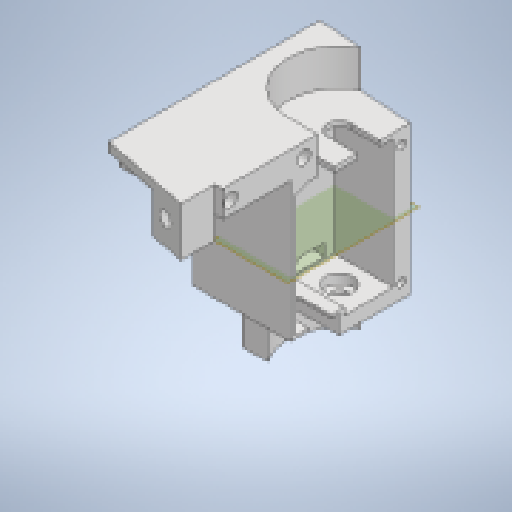
# Autodesk Inventor part: montaz_osi
Saved by Autodesk Inventor 2023.5 (Build 275446000, 446)
## iProperties
Created: 2025-03-26
Part Number: montaz_osi
Material: Ogólny
Document SubType Name: Modeling
Designer: kamil
Density: 1 g/cm^3
Appearance: Domyślna
Author: kamil
Autodesk Inventor part; units mm, degrees
ref_plane "YZ Plane" through (0, 0, 0) normal (1, 0, 0) x (0, 1, 0)
ref_plane "XZ Plane" through (0, 0, 0) normal (0, 1, 0) x (-1, 0, 0)
ref_plane "XY Plane" through (0, 0, 0) normal (0, 0, 1) x (1, 0, 0)
sketch "Szkic1" plane through (0, 0, 0) normal (0, 1, 0) x (-1, 0, 0)
  circle A0 centre (0, 0) radius 1.6
  line L0 (6, 6) -> (-6, 6)
  line L1 (-6, 6) -> (-6, -6)
  line L2 (-6, -6) -> (6, -6)
  line L3 (6, -6) -> (6, 6)
  line L4 (6, 6) -> (-6, -6) construction
  line L5 (-6, 6) -> (6, -6) construction
  dimension "d0" = 3.2
  dimension "d1" = 6
  dimension "d2" = 6
  constraints: 12 end point, 2 midpoint, 2 parallel, 1 centre point, 1 coincident, 1 horizontal, 1 perpendicular
  measures "d0" diameter of A0
  measures "d1" distance from line of L1 point (0, 0)
  measures "d2" distance from line of L2 point (0, 0)
extrude "Wyciągnięcie proste1" add sketch "Szkic1" along normal blind 1
sketch "Szkic2" plane through (0, 1, 0) normal (0, 1, 0) x (1, 0, 0)
  circle A0 centre (0, 0) radius 1.6 projected
  circle A1 centre (0, 0) radius 2.85
  line L0 (6, -6) -> (6, 6) projected
  line L1 (6, 6) -> (-6, 6) projected
  line L2 (-6, 6) -> (-6, -6) projected
  line L3 (-6, -6) -> (6, -6) projected
  circle A2 centre (0, 0) radius 1.6 projected
  dimension "d5" = 5.7
  constraints: 1 centre point, 1 coincident
  measures "d5" diameter of A1
extrude "Wyciągnięcie proste2" add sketch "Szkic2" along normal blind 2 contours L3 L2 L1 L0
sketch "Szkic3" plane through (-6, 0, 6) normal (0, 0, 1) x (1, 0, 0)
  line L0 (0, 0) -> (12, 0) projected
  line L1 (12, 0) -> (12, 3) projected
  line L2 (0, 3) -> (12, 3) projected
  line L3 (0, 0) -> (0, 3) projected
  point P0 (6, 0)
extrude "Wyciągnięcie proste3" cut sketch "Szkic3" against normal blind 1
sketch "Szkic4" plane through (-6, 0, -6) normal (-1, 0, 0) x (0, 0, 1)
  line L0 (21, 13.4099) -> (21, 27.4099) projected
  line L1 (1, 6.4099) -> (1, 20.4099) projected
  line L2 (11, 0) -> (11, 3) projected
  line L3 (0, 3) -> (11, 3) projected
  line L4 (0, 0) -> (0, 3) projected
  line L5 (0, 0) -> (11, 0) projected
  line L6 (20, 4.4099) -> (12, 4.4099) projected
  line L7 (2, 29.4099) -> (10, 29.4099) projected
  line L8 (1, 6.4099) -> (1, 3)
  line L9 (0, 3) -> (11, 3) projected
  line L10 (11, 3) -> (11, 4.4099)
  line L11 (11, 4.4099) -> (12, 4.4099)
  line L12 (1, 20.4099) -> (1, 29.4099)
  line L13 (1, 29.4099) -> (2, 29.4099)
  line L14 (1, 29.4099) -> (-2.5, 29.4099)
  line L15 (-2.5, 29.4099) -> (-2.5, 0)
  line L16 (11, 0) -> (0, 0) projected
  line L17 (-2.5, 0) -> (0, 0)
  line L18 (21, 13.4099) -> (21, 4.4099)
  line L19 (21, 4.4099) -> (20, 4.4099)
  line L20 (10, 29.4099) -> (11, 29.4099)
  line L21 (20.8, 28.4099) -> (11.2, 28.4099) projected
  line L22 (11, 29.4099) -> (11, 28.4099)
  line L23 (11, 28.4099) -> (11.2, 28.4099)
  line L24 (21, 27.4099) -> (21, 28.4099)
  line L25 (21, 28.4099) -> (20.8, 28.4099)
  point P0 (6, 0)
  dimension "d10" = 3.5
  constraints: 30 end point, 7 perpendicular, 4 point on line, 4 vertical, 1 collinear, 1 horizontal
  measures "d10" distance between parallel lines of L15 L1
extrude "Wyciągnięcie proste4" add sketch "Szkic4" along normal blind 2
sketch "Szkic5" plane through (-6, 0, -6) normal (1, 0, 0) x (0, 0, -1)
  line L0 (2.5, 29.4099) -> (2.5, 0) projected
  line L1 (-11, 29.4099) -> (2.5, 29.4099) projected
  line L2 (2.5, 0) -> (0, 0) projected
  line L3 (-11, 3) -> (0, 3) projected
  line L4 (-1, 21.4099) -> (-1, 20.4099) projected
  line L5 (-1, 28.4099) -> (-1, 29.4099) projected
  line L6 (-1, 21.4099) -> (-1, 28.4099)
  line L7 (-1, 20.4099) -> (-1, 0)
  line L8 (2.5, 0) -> (-11, 0) projected
  point P0 (-6, 0)
  constraints: 4 end point, 2 point on line, 1 vertical
extrude "Wyciągnięcie proste5" add sketch "Szkic5" along normal up to surface (12 mm away)
sketch "Szkic6" plane through (-8, 0, -6) normal (-1, 0, 0) x (0, 0, 1)
  line L0 (21, 4.4099) -> (21, 28.4099) projected
  line L1 (21, 4.4099) -> (22, 4.4099)
  line L2 (22, 4.4099) -> (22, 28.4099)
  line L3 (22, 28.4099) -> (21, 28.4099)
  line L4 (21, 28.4099) -> (21, 4.4099)
  line L5 (22, 31.9429) -> (22, -6.0571) projected
  point P0 (6, 0)
  dimension "d18" = 1
  constraints: 8 end point, 2 parallel, 1 horizontal, 1 perpendicular
  measures "d18" distance between parallel lines of L2 L0
extrude "Wyciągnięcie proste6" add sketch "Szkic6" against normal up to surface (14 mm away)
sketch "Szkic7" plane through (-8, 0, -6) normal (-1, 0, 0) x (0, 0, 1)
  line L0 (11, 0) -> (11, 4.4099) projected
  line L1 (11, 4.4099) -> (22, 4.4099) projected
  line L2 (22, 4.4099) -> (22, 28.4099) projected
  line L3 (22, 28.4099) -> (11, 28.4099) projected
  line L4 (11, 28.4099) -> (11, 29.4099) projected
  line L5 (11, 29.4099) -> (-2.5, 29.4099) projected
  line L6 (-2.5, 29.4099) -> (-2.5, 0) projected
  line L7 (-2.5, 0) -> (11, 0) projected
  line L8 (11, 28.4099) -> (22, 28.4099)
  line L9 (22, 28.4099) -> (22, 29.4099)
  line L10 (22, 29.4099) -> (11, 29.4099)
  line L11 (11, 29.4099) -> (11, 28.4099)
  line L12 (22, 4.4099) -> (22, 28.4099) projected
  point P0 (6, 0)
  constraints: 8 end point, 2 collinear, 2 parallel, 1 horizontal, 1 perpendicular
extrude "Wyciągnięcie proste7" add sketch "Szkic7" against normal up to surface (2 mm away) contours L3 L4 L10 L9
sketch "Szkic8" plane through (-6, 0, -6) normal (1, 0, 0) x (0, 0, -1)
  line L0 (-22, 28.4099) -> (-21, 28.4099) projected
  line L1 (-1, 29.4099) -> (-22, 29.4099) projected
  line L2 (-21, 4.4099) -> (-21, 28.4099) projected
  line L3 (-22, 29.4099) -> (-22, 28.4099) projected
  line L4 (-21, 28.4099) -> (-22, 28.4099)
  line L5 (-22, 28.4099) -> (-22, 29.4099)
  line L6 (-22, 29.4099) -> (-21, 29.4099)
  line L7 (-21, 29.4099) -> (-21, 28.4099)
  point P0 (-6, 0)
  constraints: 8 end point, 2 parallel, 1 horizontal, 1 perpendicular
extrude "Wyciągnięcie proste8" add sketch "Szkic8" along normal up to surface (12 mm away)
sketch "Szkic9" plane through (-8, 0, -6) normal (-1, 0, 0) x (0, 0, 1)
  line L0 (22, 29.4099) -> (-2.5, 29.4099) projected
  line L1 (22, 4.4099) -> (22, 29.4099) projected
  line L2 (16, 37.9429) -> (16, 29.9429) projected
  line L3 (16, 29.4099) -> (16, 29.9429)
  line L4 (22, 4.4099) -> (22, 29.4099) projected
  line L5 (22, 29.4099) -> (22, 37.9429)
  line L6 (22, 37.9429) -> (16, 37.9429)
  line L7 (16.5, 29.4099) -> (16.5, 29.9429)
  line L8 (16.5, 29.9429) -> (16.5, 37.4429)
  line L9 (16.5, 37.4429) -> (21.5, 37.4429)
  line L10 (21.5, 37.4429) -> (21.5, 29.4099)
  line L11 (21.5, 37.4429) -> (22, 37.4429)
  line L12 (16.5, 37.4429) -> (16.5, 37.9429)
  point P0 (6, 0)
  dimension "d23" = 0.5
  constraints: 18 end point, 4 perpendicular, 3 point on line, 2 vertical, 3 other
  measures "d23" distance between parallel lines of L6 L9
extrude "Wyciągnięcie proste9" add sketch "Szkic9" against normal up to surface (2 mm away) contours L0 L10 L11 L5 | L0 L7 L8 L9 L10 | L11 L9 L12 L6 L5
sketch "Szkic10" plane through (-6, 0, -6) normal (1, 0, 0) x (0, 0, -1)
  line L0 (-13.5, 29.9099) -> (-18.5, 29.9099) projected
  line L1 (-21, 4.4099) -> (-21, 29.4099) projected
  line L2 (-11, 4.4099) -> (-21, 4.4099) projected
  line L3 (-11, 3) -> (-11, 4.4099) projected
  line L4 (-1, 3) -> (-11, 3) projected
  line L5 (-1, 3) -> (-1, 29.4099) projected
  line L6 (-1, 29.4099) -> (-16.5, 29.4099) projected
  line L7 (-16.5, 29.4099) -> (-16.5, 37.9429) projected
  line L8 (-16.5, 37.9429) -> (-22, 37.9429) projected
  line L9 (-22, 37.9429) -> (-22, 29.4099) projected
  line L10 (-21, 29.4099) -> (-22, 29.4099) projected
  line L11 (-13.5, 30.4099) -> (-18.5, 30.4099)
  line L12 (-18.5, 30.4099) -> (-21, 29.4099)
  line L13 (-21, 29.4099) -> (-22, 29.4099) projected
  line L14 (-22, 29.4099) -> (-21, 29.4099)
  point P0 (-6, 0)
  point P1 (-16.5, 30.4099)
  dimension "d26" = 0.5
  constraints: 6 end point, 2 equal length, 1 vertical alignment
  measures "d26" distance between parallel lines of L0 L11
extrude "Wyciągnięcie proste10" add sketch "Szkic10" along normal up to surface (12 mm away) contours L10 L9 L8 L7 L11 L12
sketch "Szkic11" plane through (-8, 37.9429, 16) normal (0, 1, 0) x (1, 0, 0)
  circle A0 centre (8, 16) radius 10 projected
  circle A1 centre (8, 16) radius 10.5
  line L0 (0, 5.5) -> (14, 5.5) projected
  line L1 (0, 5.5) -> (2, 5.5) projected
  line L2 (2, 21) -> (2, 5.5) projected
  line L3 (2, 21) -> (14, 21) projected
  line L4 (14, 21) -> (14, 24.5) projected
  line L5 (14, 24.5) -> (0, 24.5) projected
  line L6 (0, 5.5) -> (0, 24.5) projected
  point P0 (8, 16)
  point P1 (8, 5.5)
  point P2 (0, 9.1993)
  constraints: 1 centre point, 1 tangent
extrude "Wyciągnięcie proste11" add sketch "Szkic11" against normal up to surface (7.533 mm away) contours L2 L0 L6 A1 | A1 L0 L2
sketch "Szkic12" plane through (-6, 30.4099, 10.5) normal (0, -1, 0) x (1, 0, 0)
  line L0 (0, -15.5) -> (0, 0) projected
  line L1 (-2, 0) -> (-2, -19) projected
  arc A0 (6, 0) -> (-2, -3.6993) centre (6, -10.5) ccw projected
  line L2 (-2, 0) -> (0, 0) projected
  point P0 (6, -10.5)
  point P1 (0, -1.8832)
extrude "Wyciągnięcie proste12" add sketch "Szkic12" along normal up to surface (1 mm away)
sketch "Szkic13" plane through (-6, 0, 5) normal (0, 0, 1) x (1, 0, 0)
  line L0 (12, 0) -> (-2, 0) projected
  line L1 (12, 3) -> (12, 0) projected
  line L2 (0, 3) -> (12, 3) projected
  line L3 (0, 3) -> (0, 4.4099) projected
  line L4 (0, 4.4099) -> (-2, 4.4099) projected
  line L5 (-2, 0) -> (-2, 4.4099) projected
  line L6 (12, 3) -> (12, 0) projected
  line L7 (-2, 0) -> (-2, 4.4099) projected
  line L8 (12, 0) -> (-2, 0)
  line L9 (-2, 0) -> (-2, 4.4099)
  line L10 (-2, 4.4099) -> (12, 4.4099)
  line L11 (12, 4.4099) -> (12, 0)
  point P0 (6, 0)
  constraints: 8 end point, 2 parallel, 1 horizontal, 1 perpendicular
extrude "Wyciągnięcie proste13" add sketch "Szkic13" along normal blind 1
sketch "Szkic14" plane through (-8, 4.4099, 16) normal (0, -1, 0) x (1, 0, 0)
  line L0 (0, -10) -> (0, 0) projected
  line L1 (0, 0) -> (14, 0) projected
  line L2 (14, -10) -> (2, -10) projected
  line L3 (0, -10) -> (2, -10) projected
  circle A0 centre (8, -6) radius 1.95 projected
  circle A1 centre (8, -6) radius 2.35
  line L4 (14, -10) -> (14, -2) projected
  line L5 (14, -1) -> (14, 0) projected
  line L6 (14, -2) -> (14, -1)
  line L7 (8, -8.35) -> (14, -8.35)
  line L8 (8, -3.65) -> (14, -3.65)
  line L9 (14, -5.5) -> (14, -3.5) projected
  point P0 (8, -16)
  point P1 (14, -3.65)
  dimension "d36" = 0.4
  constraints: 6 end point, 2 perpendicular, 2 point on circle, 2 point on line, 2 tangent, 1 centre point, 1 vertical
  measures "d36" radial gap between concentric circles of A0 A1
extrude "Wyciągnięcie proste14" add sketch "Szkic14" along normal blind 0.6 contours L0 L1 L5 L6 L4 L8 A1 L7 L2 L3
sketch "Szkic15" plane through (-8, 29.4099, -8.5) normal (0, 1, 0) x (1, 0, 0)
  circle A0 centre (8, -8.5) radius 1.95 projected
  circle A1 centre (8, -8.5) radius 2.35
  line L0 (0, -15.3007) -> (0, 0) projected
  line L1 (14, 0) -> (0, 0) projected
  line L2 (3, -13.5) -> (13, -13.5) projected
  line L3 (3, -15.5) -> (13, -15.5)
  line L4 (3, -15.5) -> (0, -15.5)
  line L5 (0, -15.5) -> (0, -15.3007)
  line L6 (14, -18.5) -> (14, 0) projected
  line L7 (13, -15.5) -> (14, -15.5)
  line L8 (13, -13.5) -> (14, -13.5)
  line L9 (8, -8.5) -> (8, -10.85)
  line L10 (8, -10.85) -> (14, -10.85)
  line L11 (8, -6.15) -> (14, -6.15)
  point P0 (8, -8.5)
  dimension "d39" = 0.4
  dimension "d40" = 2
  constraints: 16 end point, 5 perpendicular, 5 point on line, 2 point on circle, 1 centre point, 1 horizontal, 1 parallel, 1 tangent, 1 vertical
  measures "d39" radial gap between concentric circles of A0 A1
  measures "d40" distance between parallel lines of L2 L3
extrude "Wyciągnięcie proste15" add sketch "Szkic15" along normal blind 1 contours A1 L10 L6 L7 L3 L4 L5 L0 L1 L11
sketch "Szkic16" plane through (-7.8262, 29.4099, 7) normal (0, 1, 0) x (1, 0, 0)
  line L0 (1.8262, 0) -> (0, 0) projected
  arc A0 (0, 0) -> (1.8262, -1.6168) centre (7.8262, 7) ccw projected
  line L1 (1.8262, 0) -> (1.8262, -1.6168) projected
  point P0 (7.8262, 7)
extrude "Wyciągnięcie proste16" add sketch "Szkic16" along normal up to surface (1 mm away)
sketch "Szkic17" plane through (-8, 30.4099, -8.5) normal (0, 1, 0) x (1, 0, 0)
  circle A0 centre (8, -8.5) radius 10 projected
  circle A1 centre (8, -8.5) radius 10 projected
  circle A2 centre (8, -8.5) radius 9.5
  line L0 (14, -6.15) -> (14, 0) projected
  line L1 (14, 0) -> (0, 0) projected
  point P0 (8, -8.5)
  point P1 (12.2426, 0)
  point P2 (14, -1.1345)
  dimension "d45" = 0.5
  constraints: 1 centre point
  measures "d45" radial gap between concentric circles of A0 A2
sketch "Szkic18" plane through (6, 37.9429, 16) normal (1, 0, 0) x (0, 0, -1)
  line L0 (1, -8.533) -> (1, -33.533) projected
  line L1 (3.5, -7.533) -> (1, -8.533) projected
  line L2 (5.5, -7.533) -> (3.5, -7.533) projected
  line L3 (5.5, 0) -> (5.5, -7.533) projected
  line L4 (0, 0) -> (5.5, 0) projected
  line L5 (0, 0) -> (0, -34.133) projected
  line L6 (3.65, -34.133) -> (0, -34.133) projected
  line L7 (3.65, -33.533) -> (3.65, -34.133) projected
  line L8 (3.65, -33.533) -> (1, -33.533) projected
  point P0 (16, -37.9429)
  point P1 (2.75, -2.75)
  point P2 (2.75, 0)
  dimension "d48" = 2.75
  constraints: 1 midpoint, 1 vertical alignment
  measures "d48" distance from line of L4 point (2.75, -2.75)
hole "Otwór1" at (6, 35.1929, 13.25) direction (-1, 0, 0) diameter 2.8 end through all
ref_plane "Płaszczyzna konstrukcyjna1" through (0, 15.2049, 0) normal (0, -1, 0) x (1, 0, 0)
sketch "Szkic20" plane through (6, 3, 5) normal (1, 0, 0) x (0, 0, -1)
  line L0 (0, 0) -> (10, 0) projected
  line L1 (0, 0) -> (0, 1.4099) projected
  line L2 (0, 1.4099) -> (-2.65, 1.4099) projected
  line L3 (-2.65, 1.4099) -> (-2.65, 0.8099) projected
  line L4 (-1, 0.8099) -> (-2.65, 0.8099) projected
  line L5 (-1, -3) -> (-1, 0.8099) projected
  line L6 (-1, -3) -> (13.5, -3) projected
  line L7 (13.5, 27.4099) -> (13.5, -3) projected
  line L8 (7.35, 27.4099) -> (13.5, 27.4099) projected
  line L9 (7.35, 26.4099) -> (7.35, 27.4099) projected
  line L10 (7.35, 26.4099) -> (10, 26.4099) projected
  line L11 (10, 0) -> (10, 26.4099) projected
  line L12 (10, 26.4099) -> (13.5, 26.4099)
  line L13 (13.5, 27.4099) -> (13.5, -3) projected
  line L14 (0, 0) -> (10, 0) projected
  line L15 (10, 0) -> (10, -3)
  line L16 (-1, -3) -> (13.5, -3) projected
  line L17 (11.75, 26.4099) -> (11.75, -3)
  point P0 (5, -3)
  point P1 (11.75, 24.4099)
  point P2 (11.75, 0)
  dimension "d64" = 3
  dimension "d65" = 3
  constraints: 6 end point, 5 point on line, 3 perpendicular, 1 midpoint
  measures "d64" distance from line of point (11.75, 0) L6
  measures "d65" distance from line of L8 point (11.75, 24.41)
hole "Otwór3" at (6, 27.4099, -6.75) at (6, 3, -6.75) direction (-1, 0, 0) diameter 1.7 end through all
sketch "Szkic21" plane through (6, 37.9429, 16) normal (1, 0, 0) x (0, 0, -1)
  line L0 (-0.5, -5.5) -> (-13.5, -5.5) projected
  line L1 (-13.5, -44.5) -> (-0.5, -44.5) projected
  line L2 (-24, 0) -> (26, 0) projected
  line L3 (0, 0) -> (0, -34.133) projected
  line L4 (0, -5.5) -> (-14, -5.5)
  line L5 (-14, -5.5) -> (-14, 0)
  line L6 (-14, 0) -> (0, 0)
  line L7 (0, 0) -> (0, -5.5)
  line L8 (-14, -6) -> (-14, -44) projected
  point P0 (16, -37.9429)
  point P1 (-13.5, -5.5)
  constraints: 8 end point, 2 parallel, 2 point on line, 1 collinear, 1 horizontal, 1 perpendicular
extrude "Wyciągnięcie proste18" add sketch "Szkic21" against normal up to surface (14 mm away)
sketch "Szkic22" plane through (6, 30.4099, 10.5) normal (1, 0, 0) x (0, 0, -1)
  line L0 (-19.5, 1.533) -> (-19.5, -36.467) projected
  line L1 (-19.5, 2.033) -> (-5.5, 2.033) projected
  line L2 (-19.5, 7.533) -> (-19.5, 2.033) projected
  line L3 (-19.5, 1.533) -> (-19.5, 2.033)
  line L4 (-29.5, 7.533) -> (20.5, 7.533) projected
  line L5 (-29.5, -42.467) -> (-29.5, 7.533) projected
  line L6 (20.5, -42.467) -> (-29.5, -42.467) projected
  line L7 (20.5, 7.533) -> (20.5, -42.467) projected
  line L8 (-27.5, -40.467) -> (18.5, -40.467) projected
  line L9 (-27.5, 5.533) -> (-27.5, -40.467) projected
  line L10 (18.5, 5.533) -> (-27.5, 5.533) projected
  line L11 (18.5, -40.467) -> (18.5, 5.533) projected
  line L12 (-20.5, 7.533) -> (-20.5, -2.467)
  line L13 (-20.5, -2.467) -> (-19.5, -2.467)
  point P0 (10.5, -30.4099)
  point P1 (-20, -2.467)
  dimension "d75" = 1
  dimension "d76" = 10
  constraints: 6 end point, 2 point on line, 2 vertical, 1 midpoint, 1 perpendicular
  measures "d75" distance between parallel lines of L0 L12
  measures "d76" distance from line of L4 point (-20, -2.467)
extrude "Wyciągnięcie proste19" add sketch "Szkic22" against normal up to surface (14 mm away) contours L0 L13 L12 L10 L2 L3 | L10 L12 L4 L2
sketch "Szkic23" plane through (6, 30.4099, 10.5) normal (1, 0, 0) x (0, 0, -1)
  circle A0 centre (-2.75, 4.783) radius 1.4 projected
  line L0 (-4.5, -1) -> (-4.5, -26) projected
  line L1 (-2, 0) -> (-4.5, -1) projected
  line L2 (0, 0) -> (-2, 0) projected
  line L3 (0, 7.533) -> (0, 0) projected
  line L4 (0, 7.533) -> (-20.5, 7.533) projected
  line L5 (-20.5, 7.533) -> (-20.5, -2.467) projected
  line L6 (-20.5, -2.467) -> (-19.5, -2.467) projected
  line L7 (-19.5, -2.467) -> (-19.5, 2.033) projected
  line L8 (-19.5, 2.033) -> (-5.5, 2.033) projected
  line L9 (-5.5, 2.033) -> (-5.5, -26.6) projected
  line L10 (-1.85, -26.6) -> (-5.5, -26.6) projected
  line L11 (-1.85, -26) -> (-1.85, -26.6) projected
  line L12 (-1.85, -26) -> (-4.5, -26) projected
  point P0 (10.5, -30.4099)
  point P1 (-17.75, 4.783)
  dimension "d79" = 2.75
  dimension "d80" = 2.75
  constraints: 1 horizontal alignment
  measures "d79" distance from line of L4 point (-17.75, 4.783)
  measures "d80" distance from line of L5 point (-17.75, 4.783)
hole "Otwór4" at (6, 35.1929, 28.25) direction (-1, 0, 0) diameter 2.8 end through all
sketch "Szkic24" plane through (-8, 0, -6) normal (-1, 0, 0) x (0, 0, 1)
  circle A0 centre (17.5, 35.4429) radius 1.3 projected
  line L0 (37, 37.9429) -> (12.8007, 37.9429) projected
  line L1 (12.8007, 37.9429) -> (12.8007, 30.4099) projected
  line L2 (22.1993, 32.9429) -> (12.8007, 32.9429)
  line L3 (12.8007, 32.9429) -> (12.8007, 37.9429)
  line L4 (12.8007, 37.9429) -> (22.1993, 37.9429)
  line L5 (22.1993, 37.9429) -> (22.1993, 32.9429)
  line L6 (22.1993, 32.9429) -> (12.8007, 37.9429) construction
  line L7 (12.8007, 32.9429) -> (22.1993, 37.9429) construction
  line L8 (22, 32.4429) -> (22.1993, 32.9429)
  line L9 (36, 32.4429) -> (22, 32.4429) projected
  line L10 (22, 32.4429) -> (12.8007, 32.4429)
  point P0 (6, 0)
  constraints: 16 end point, 2 midpoint, 2 parallel, 2 perpendicular, 1 horizontal, 1 point on line
ref_plane "Płaszczyzna konstrukcyjna2" through (-15.1166, -12.0571, -10) normal (1, 0, 0) x (0, 1, 0)
ref_plane "Płaszczyzna konstrukcyjna3" through (-14, -12.0571, -10) normal (1, 0, 0) x (0, 1, 0)
extrude "Wyciągnięcie proste20" add sketch "Szkic24" along normal up to surface (6 mm away)
sketch "Szkic26" plane through (-8, 0, -6) normal (-1, 0, 0) x (0, 0, 1)
  line L0 (22, 32.4429) -> (12.8007, 32.4429) projected
  line L1 (12.8007, 32.4429) -> (12.8007, 30.4099) projected
  line L2 (-2.5, 30.4099) -> (12.8007, 30.4099) projected
  line L3 (-2.5, 0) -> (-2.5, 30.4099) projected
  line L4 (-2.5, 0) -> (12, 0) projected
  line L5 (12, 3.8099) -> (12, 0) projected
  line L6 (22, 3.8099) -> (12, 3.8099) projected
  line L7 (22, 3.8099) -> (22, 32.4429) projected
  circle A0 centre (-0.75, 27.4099) radius 0.85 projected
  circle A1 centre (-0.75, 3) radius 0.85 projected
  point P0 (6, 0)
extrude "Wyciągnięcie proste21" add sketch "Szkic26" along normal up to surface (6 mm away) contours L7 L6 L5 L4 L3 L2 L1 L0 | A0 | A1
sketch "Szkic27" plane through (-14, 0, -8.5) normal (-1, 0, 0) x (0, 0, 1)
  circle A0 centre (20, -9.5571) radius 1.3 projected
  line L0 (-1.5, -12.0571) -> (48.5, -12.0571) projected
  line L1 (24.5, 3.8099) -> (24.5, 32.4429) projected
  line L2 (0, 30.4099) -> (0, 0) projected
  line L3 (0, 0) -> (14.5, 0) projected
  line L4 (14.5, 0) -> (14.5, 3.8099) projected
  line L5 (14.5, 3.8099) -> (24.5, 3.8099) projected
  line L6 (15.3007, 37.9429) -> (15.3007, 30.4099) projected
  line L7 (15.3007, 0) -> (15.3007, -12.0571)
  line L8 (24.5, 32.4429) -> (24.5, 3.8099) projected
  line L9 (24.5, 3.8099) -> (24.5, -12.0571)
  line L10 (14.5, 0) -> (15.3007, 0)
  point P0 (8.5, 0)
  constraints: 6 end point, 2 collinear, 2 point on line, 1 horizontal, 1 perpendicular, 1 vertical
extrude "Wyciągnięcie proste22" add sketch "Szkic27" against normal blind 4
fillet "Zaokrąglenie1" radius 5 1 edges at (-10, 3.8099, 11)
sketch "Szkic28" plane through (0, 0, 0) normal (0, -1, 0) x (1, 0, 0)
  arc A0 (0, 10.5) -> (-8, 6.8007) centre (0, 0) ccw projected
  circle A1 centre (0, 0) radius 1.6 projected
  line L0 (6, 6) -> (6, -8.5) projected
  line L1 (6, 6) -> (-9.8563, 6) projected
  line L2 (-9.8563, 6.8007) -> (-9.8563, 6) projected
  line L3 (-14, 6.8007) -> (-9.8563, 6.8007) projected
  line L4 (-14, -8.5) -> (-14, 6.8007) projected
  line L5 (6, -8.5) -> (-14, -8.5) projected
  circle A2 centre (0, 0) radius 10.5
  point P0 (-6.1644, -8.5)
  point P1 (-8.6168, 6)
  constraints: 1 centre point, 1 coincident, 1 concentric
extrude "Wyciągnięcie proste23" add sketch "Szkic28" along normal up to surface (12.0571 mm away) contours A2 L5 L4 L3 L2 L1
sketch "Szkic29" plane through (-8, 30.4099, -8.5) normal (0, 1, 0) x (1, 0, 0)
  arc A0 (0, -15.3007) -> (2, -17.1168) centre (8, -8.5) ccw projected
  line L0 (2, -15.5) -> (2, -17.1168) projected
  line L1 (2, -15.5) -> (14, -15.5) projected
  line L2 (14, -15.5) -> (14, -10.85) projected
  line L3 (14, -10.85) -> (8, -10.85) projected
  arc A1 (8, -6.15) -> (8, -10.85) centre (8, -8.5) ccw projected
  line L4 (8, -6.15) -> (14, -6.15) projected
  line L5 (14, -6.15) -> (14, 0) projected
  line L6 (14, 0) -> (-6, 0) projected
  line L7 (-6, -15.3007) -> (-6, 0) projected
  line L8 (0, -15.3007) -> (-6, -15.3007) projected
  arc A2 (0, -15.3007) -> (8, -19) centre (8, -8.5) ccw projected
  circle A3 centre (8, -8.5) radius 10.5
  point P0 (8, -8.5)
  point P1 (1.8356, 0)
  constraints: 1 coincident, 3 other
extrude "Wyciągnięcie proste24" add sketch "Szkic29" along normal up to surface (7.533 mm away) contours L8 L7 L6 A3
sketch "Szkic30" plane through (6, 3, 5) normal (1, 0, 0) x (0, 0, -1)
  line L0 (-1, 0.8099) -> (-11, 0.8099)
  line L1 (-11, 0.8099) -> (-11, -15.0571)
  line L2 (-11, -15.0571) -> (-1, -15.0571)
  line L3 (-1, -15.0571) -> (-1, 0.8099)
  point P0 (5, -3)
  constraints: 8 end point, 2 parallel, 1 horizontal, 1 perpendicular
extrude "Wyciągnięcie proste25" cut sketch "Szkic30" against normal through all
sketch "Szkic31" plane through (0, 37.9429, 10.5) normal (0, 1, 0) x (1, 0, 0)
  line L0 (-8, -20.5) -> (-8, -5.6993) projected
  line L1 (6, -20.5) -> (-8, -20.5) projected
  line L2 (6, 0) -> (6, -20.5) projected
  line L3 (0, 0) -> (6, 0) projected
  arc A0 (-6.1644, 19) -> (0, 0) centre (0, 10.5) ccw projected
  line L4 (-14, 19) -> (-6.1644, 19) projected
  line L5 (-14, -5.6993) -> (-14, 19) projected
  line L6 (-8, -5.6993) -> (-14, -5.6993) projected
  line L7 (10, -27.4622) -> (-26.4275, -20.3419) projected
  line L8 (6, -26.6803) -> (6, 0.5) projected
  line L9 (-4.0145, -24.7228) -> (-4.0145, -20.5)
  line L10 (6, -20.5) -> (-8, -20.5) projected
  point P0 (0, 10.5)
  constraints: 2 end point, 2 point on line, 1 perpendicular
extrude "Wyciągnięcie proste26" add sketch "Szkic31" against normal up to surface (5.5 mm away) contours L1 L8 L7 L9
sketch "Szkic32" plane through (0, 37.9429, 10.5) normal (0, 1, 0) x (1, 0, 0)
  line L0 (-8, -20.5) -> (-8, -5.6993) projected
  line L1 (-4.0145, -20.5) -> (-4.0145, -24.7228) projected
  line L2 (-4.0145, -20.5) -> (-8, -20.5) projected
  line L3 (10, -27.4622) -> (-26.4275, -20.3419) projected
  line L4 (-14, 0) -> (-14, -21.9466) projected
  line L5 (-14, -21.9466) -> (-14, -22.771)
  line L6 (-8, -5.6993) -> (-14, -5.6993) projected
  point P0 (0, 10.5)
  constraints: 2 end point, 1 point on line, 1 vertical
extrude "Wyciągnięcie proste27" add sketch "Szkic32" against normal blind 1.8
sketch "Szkic33" plane through (-8, 0, -6) normal (-1, 0, 0) x (0, 0, 1)
  line L0 (37, 36.1429) -> (35.2783, 36.1429) projected
  arc A0 (33.2217, 36.1429) -> (35.2783, 36.1429) centre (34.25, 35.1929) ccw projected
  line L1 (33.2217, 36.1429) -> (22.1993, 36.1429) projected
  line L2 (22.1993, 36.1429) -> (22.1993, 32.9429) projected
  line L3 (22.1993, 32.9429) -> (22, 32.4429) projected
  line L4 (36, 32.4429) -> (22, 32.4429) projected
  line L5 (36, 27.9429) -> (36, 32.4429) projected
  line L6 (37, 27.9429) -> (36, 27.9429) projected
  line L7 (37, 36.1429) -> (37, 27.9429) projected
  line L8 (37, 32.4429) -> (36, 32.4429)
  point P0 (6, 0)
  constraints: 2 end point, 1 perpendicular, 1 point on line
extrude "Wyciągnięcie proste28" cut sketch "Szkic33" against normal up to surface (3.9855 mm away) contours L7 L6 L5 L8
sketch "Szkic34" plane through (6, 32.4429, 31) normal (0, -1, 0) x (1, 0, 0)
  line L0 (0, 0) -> (0, 6.1803) projected
  line L1 (0, 6.1803) -> (-10.0145, 4.2228) projected
  line L2 (-10.0145, 4.2228) -> (-10.0145, 0) projected
  line L3 (0, 0) -> (-10.0145, 0) projected
  point P0 (-6, -31)
extrude "Wyciągnięcie proste29" add sketch "Szkic34" along normal up to surface (4.5 mm away)
sketch "Szkic35" plane through (-14, 3.8099, 16) normal (-1, 0, 0) x (0, 0, 1)
  line L0 (0, 28.633) -> (15, 28.633) projected
  line L1 (15, 32.333) -> (15, 28.633) projected
  line L2 (15, 32.333) -> (13.2783, 32.333) projected
  arc A0 (11.2217, 32.333) -> (13.2783, 32.333) centre (12.25, 31.383) ccw projected
  line L3 (11.2217, 32.333) -> (0.1993, 32.333) projected
  line L4 (0.1993, 32.333) -> (0.1993, 29.133) projected
  line L5 (0.1993, 29.133) -> (0, 28.633) projected
  line L6 (17.271, 32.333) -> (0.1993, 32.333) projected
  point P0 (-16, -3.8099)
extrude "Wyciągnięcie proste30" add sketch "Szkic35" against normal up to surface (6 mm away)
sketch "Szkic36" plane through (-4.0145, 27.9429, 30) normal (-1, 0, 0) x (0, 0, 1)
  line L0 (5.2228, 8.2) -> (1, 8.2) projected
  line L1 (1, 4.5) -> (1, 8.2) projected
  line L2 (0, 4.5) -> (1, 4.5) projected
  line L3 (0, 0) -> (0, 4.5) projected
  line L4 (0, 0) -> (5.2228, 0) projected
  line L5 (5.2228, 8.2) -> (5.2228, 0) projected
  line L6 (5.2228, 8.2) -> (1, 8.2) projected
  line L7 (5.2228, 8.2) -> (10.0284, 8.2)
  line L8 (10.0284, 8.2) -> (10.0284, 0)
  line L9 (10.0284, 0) -> (5.2228, 0)
  line L10 (5.2228, 0) -> (5.2228, 8.2)
  point P0 (-30, -27.9429)
  point P1 (5.2228, 0)
  constraints: 8 end point, 2 parallel, 1 horizontal, 1 perpendicular
extrude "Wyciągnięcie proste31" cut sketch "Szkic36" against normal blind 1
sketch "Szkic37" plane through (6, 27.9429, 37.1803) normal (-0.1918332, 0, 0.9814276) x (0.9814276, 0, 0.1918332)
  line L0 (0, 10) -> (0, 0) projected
  line L1 (-9.1851, 8.2) -> (-9.1851, 0) projected
  line L2 (-9.1851, 0) -> (0, 0) projected
  line L3 (0, 10) -> (0, 0) projected
  line L4 (-20.3785, 10) -> (0, 10) projected
  line L5 (-20.3785, 10) -> (-20.3785, 8.2) projected
  line L6 (-20.3785, 8.2) -> (-9.1851, 8.2) projected
  point P0 (-13.021, -27.9429)
  point P1 (-5.6851, 5)
  point P2 (0, 5)
  dimension "d115" = 3.5
  constraints: 1 horizontal alignment, 1 midpoint
  measures "d115" distance from line of point (-5.685, 5) L1
hole "Otwór5" at (0.4205, 32.9429, 36.0897) direction (0.1918332, 0, -0.9814276) diameter 2.8 depth 7 tip angle 118
sketch "Szkic38" plane through (-14, 32.4429, 16) normal (-1, 0, 0) x (0, 0, 1)
  circle A0 centre (-4.5, 3) radius 1.3 projected
  circle A1 centre (-4.5, 3) radius 1.15
  point P0 (-16, -32.4429)
  dimension "d123" = 2.3
  constraints: 1 centre point, 1 coincident
  measures "d123" diameter of A1
extrude "Wyciągnięcie proste32" add sketch "Szkic38" against normal up to surface (6 mm away)
sketch "Szkic39" plane through (0, 37.9429, 10.5) normal (0, 1, 0) x (1, 0, 0)
  line L0 (-14, -22.771) -> (6, -26.6803) projected
  line L1 (6, 0) -> (6, -26.6803) projected
  line L2 (0, 0) -> (6, 0) projected
  arc A0 (-6.1644, 19) -> (0, 0) centre (0, 10.5) ccw projected
  line L3 (-14, 19) -> (-6.1644, 19) projected
  line L4 (-14, -22.771) -> (-14, 19) projected
  line L5 (6, -19.3676) -> (4.4, -19.3676) projected
  line L6 (4.4, -19.3676) -> (4.4, -26.3676) projected
  point P0 (0, 10.5)
extrude "Wyciągnięcie proste33" cut sketch "Szkic39" against normal through all contours L6 L5 L1 L0
sketch "Szkic40" plane through (-14, 32.4429, 16) normal (-1, 0, 0) x (0, 0, 1)
  line L0 (-11.9309, -3.182) -> (-9.3105, -3.182)
  line L1 (-9.3105, -3.182) -> (-9.3105, -5.2718)
  line L2 (-9.3105, -5.2718) -> (-11.9309, -5.2718)
  line L3 (-11.9309, -5.2718) -> (-11.9309, -3.182)
  line L4 (-12.0052, -33.4358) -> (-9.3894, -33.4358)
  line L5 (-9.3894, -33.4358) -> (-9.3894, -35.5938)
  line L6 (-9.3894, -35.5938) -> (-12.0052, -35.5938)
  line L7 (-12.0052, -35.5938) -> (-12.0052, -33.4358)
  line L8 (-8.8894, -32.9358) -> (-12.5052, -32.9358)
  line L9 (-12.5052, -32.9358) -> (-12.5052, -36.0938)
  line L10 (-12.5052, -36.0938) -> (-8.8894, -36.0938)
  line L11 (-8.8894, -36.0938) -> (-8.8894, -32.9358)
  line L12 (-8.8105, -2.682) -> (-12.4309, -2.682)
  line L13 (-12.4309, -2.682) -> (-12.4309, -5.7718)
  line L14 (-12.4309, -5.7718) -> (-8.8105, -5.7718)
  line L15 (-8.8105, -5.7718) -> (-8.8105, -2.682)
  point P0 (-16, -32.4429)
  dimension "d128" = 0.5
  dimension "d129" = 0.5
  constraints: 32 end point, 8 parallel, 4 perpendicular, 2 horizontal, 10 other
  measures "d128" distance between parallel lines of L4 L8
  measures "d129" distance between parallel lines of L0 L12
sketch "Szkic41" plane through (-6, 0, -6) normal (1, 0, 0) x (0, 0, -1)
  line L0 (-3.5, 3.9099) -> (-3.5, 5.4099)
  line L1 (-8.5, 3.9099) -> (-8.5, 5.4099)
  line L2 (-13.5, 29.9099) -> (-13.5, 28.4099)
  line L3 (-18.5, 29.9099) -> (-18.5, 28.4099)
  line L4 (-18.5, 29.9099) -> (-13.5, 29.9099)
  line L5 (-13.5, 29.9099) -> (-13.5, 28.4099)
  line L6 (-13.5, 28.4099) -> (-18.5, 28.4099)
  line L7 (-18.5, 28.4099) -> (-18.5, 29.9099)
  line L8 (-8.5, 5.4099) -> (-3.5, 5.4099)
  line L9 (-3.5, 5.4099) -> (-3.5, 3.9099)
  line L10 (-3.5, 3.9099) -> (-8.5, 3.9099)
  line L11 (-8.5, 3.9099) -> (-8.5, 5.4099)
  line L12 (-9, 5.9099) -> (-3, 5.9099)
  line L13 (-3, 5.9099) -> (-3, 3.4099)
  line L14 (-3, 3.4099) -> (-9, 3.4099)
  line L15 (-9, 3.4099) -> (-9, 5.9099)
  line L16 (-13.5, 27.9099) -> (-19, 27.9099)
  line L17 (-19, 27.9099) -> (-19, 30.0701)
  line L18 (-18.9005, 30.1099) -> (-13.3, 30.1099)
  line L19 (-13.3, 30.1099) -> (-13.3, 28.4099)
  line L20 (-18.9005, 30.1099) -> (-19, 30.0701)
  line L21 (-13.5, 27.9099) -> (-13.3, 27.9099)
  line L22 (-13.3, 27.9099) -> (-13.3, 28.4099)
  point P0 (-6, 0)
  dimension "d132" = 0.5
  dimension "d133" = 0.5
  dimension "d134" = 0.5
  dimension "d135" = 0.5
  dimension "d136" = 0.5
  dimension "d137" = 0.2
  constraints: 46 end point, 6 parallel, 5 perpendicular, 4 horizontal, 4 vertical, 10 other
  measures "d132" distance between parallel lines of L12 L8
  measures "d133" distance between parallel lines of L10 L14
  measures "d134" distance between parallel lines of L1 L15
  measures "d135" distance between parallel lines of L13 L0
  measures "d136" distance between parallel lines of L6 L16
  measures "d137" distance between parallel lines of L4 L18
extrude "Wyciągnięcie proste34" cut sketch "Szkic40" against normal blind 4 contours L0 L1 L2 L3 | L4 L5 L6 L7 | L11 L10 L9 L8 | L15 L14 L13 L12
extrude "Wyciągnięcie proste35" cut sketch "Szkic41" against normal blind 2 contours L10 L1 L8 L0 | L2 L6 L3 L4 | L12 L13 L14 L15 | L16 L17 L20 L18 L19 L22 L21
sketch "Szkic42" plane through (-6, 27.9099, 13) normal (0, 1, 0) x (1, 0, 0)
  line L0 (0, 5.7) -> (0, 0) projected
  line L1 (0, 5.7) -> (-2, 5.7) projected
  line L2 (-2, 5.7) -> (-2, 0) projected
  line L3 (0, 0) -> (-2, 0) projected
  point P0 (6, 13)
extrude "Wyciągnięcie proste36" cut sketch "Szkic42" against normal up to surface (1.2388 mm away)
sketch "Szkic43" plane through (-8, 26.6711, 7.3) normal (0, 1, 0) x (1, 0, 0)
  line L0 (2, 0) -> (2, -5.7) projected
  line L1 (2, 0) -> (0, 0) projected
  line L2 (0, 0) -> (0, -5.7) projected
  line L3 (0, -5.7) -> (2, -5.7) projected
  line L4 (-6, 0.1105) -> (-6, 3.7309) projected
  line L5 (-6, 0.1105) -> (-2, 0.1105) projected
  line L6 (-2, 0.1105) -> (-2, 3.7309) projected
  line L7 (-6, 3.7309) -> (-2, 3.7309) projected
  line L8 (0, -5.7) -> (-2, 0.1105)
  line L9 (2, 0) -> (0, 0) projected
  line L10 (0, 0) -> (-2, 3.7309)
  point P0 (8, 7.3)
  constraints: 4 end point
extrude "Wyciągnięcie proste37" cut sketch "Szkic43" along normal up to surface (3.0898 mm away) contours L2 L8 L6 L10
sketch "Szkic44" plane through (-6, 30.1099, 7.3) normal (0, -1, 0) x (1, 0, 0)
  line L0 (0, 5.6005) -> (0, 0) projected
  line L1 (0, 5.6005) -> (-2, 5.6005) projected
  line L2 (-2, 5.6005) -> (-2, 0) projected
  line L3 (0, 0) -> (-2, 0) projected
  line L4 (0, 5.7) -> (0, 5.6005) projected
  line L5 (0, 5.7) -> (-2, 5.7) projected
  line L6 (-2, 5.7) -> (-2, 5.6005) projected
  line L7 (0, 5.6005) -> (-2, 5.6005) projected
  point P0 (6, -7.3)
extrude "Wyciągnięcie proste38" add sketch "Szkic44" along normal up to surface (0.349 mm away)
fillet "Zaokrąglenie3" radius 2 1 edges at (-10, 28.216, 7.1895)
fillet "Zaokrąglenie4" radius 1 2 edges at (-8, 27.2905, 13) (-8, 28.8354, 13)
sketch "Szkic45" plane through (-14, 32.4429, 16) normal (-1, 0, 0) x (0, 0, 1)
  line L0 (-19, -29.033) -> (-13, -29.033) projected
  line L1 (-19, -26.533) -> (-19, -29.033) projected
  line L2 (-13, -26.533) -> (-19, -26.533) projected
  line L3 (-13, -29.033) -> (-13, -26.533) projected
  point P0 (-16, -32.4429)
extrude "Wyciągnięcie proste39" cut sketch "Szkic45" against normal through all
sketch "Szkic46" plane through (-14, 32.4429, 16) normal (-1, 0, 0) x (0, 0, 1)
  line L0 (-19, -26.533) -> (-13, -26.533) projected
  line L1 (-13, -26.533) -> (-13, -29.033) projected
  line L2 (-13, -29.033) -> (-19, -29.033) projected
  line L3 (-19, -29.033) -> (-19, -26.533) projected
  line L4 (-10, -36.0938) -> (-12.5052, -36.0938) projected
  line L5 (-12.5052, -36.0938) -> (-12.5052, -32.9358) projected
  line L6 (-12.5052, -32.9358) -> (-10, -32.9358) projected
  line L7 (-10, -32.9358) -> (-10, -28.633) projected
  line L8 (-10, -28.633) -> (0, -28.633) projected
  line L9 (0, -28.633) -> (0, 0) projected
  line L10 (0, 0) -> (15, 0) projected
  line L11 (15, 0) -> (15, 3.7) projected
  line L12 (17.271, 3.7) -> (15, 3.7) projected
  line L13 (17.271, 5.5) -> (17.271, 3.7) projected
  line L14 (17.271, 5.5) -> (-24.5, 5.5) projected
  line L15 (-24.5, 5.5) -> (-24.5, -44.5) projected
  line L16 (-24.5, -44.5) -> (-10, -44.5) projected
  line L17 (-10, -44.5) -> (-10, -36.0938) projected
  circle A0 centre (-4.5, 3) radius 1.15 projected
  line L18 (-8.8105, -5.7718) -> (-12.4309, -5.7718) projected
  line L19 (-12.4309, -5.7718) -> (-12.4309, -2.682) projected
  line L20 (-12.4309, -2.682) -> (-8.8105, -2.682) projected
  line L21 (-8.8105, -2.682) -> (-8.8105, -5.7718) projected
  line L22 (-12.5052, -36.0938) -> (-12.5052, -32.9358) projected
  line L23 (-13, -29.033) -> (-12.5052, -32.9358)
  line L24 (-10, -36.0938) -> (-12.5052, -36.0938) projected
  line L25 (-12.5052, -36.0938) -> (-15.1047, -36.0938)
  line L26 (-15.1047, -36.0938) -> (-16, -29.033)
  line L27 (-19, -29.033) -> (-13, -29.033) projected
  point P0 (-16, -32.4429)
  constraints: 6 end point, 2 midpoint, 1 parallel, 1 point on line
extrude "Wyciągnięcie proste40" cut sketch "Szkic46" against normal blind 2 contours L23 L5 L25 L26 L2
fillet "Zaokrąglenie5" radius 1 7 edges at (-12, 3.4099, 1.5) (-12, -2.0719, 3.4948) (-10, -2.0719, 3.4948) (-13, -3.6509, 0.8953) (-13, 3.4099, 0) (-10, 5.9099, 3) (-13, -0.4929, 3.4948)
sketch "Szkic47" plane through (-14, 32.4429, 16) normal (-1, 0, 0) x (0, 0, 1)
  line L0 (-12.4407, 1.8649) -> (-16.6576, 1.8649)
  line L1 (-16.6576, 1.8649) -> (-16.6576, 4.2825)
  line L2 (-16.6576, 4.2825) -> (-12.4407, 4.2825)
  line L3 (-12.4407, 4.2825) -> (-12.4407, 1.8649)
  line L4 (6.564, 2.6398) -> (-0.8394, 2.6398)
  line L5 (-0.8394, 2.6398) -> (-0.8394, 4.5479)
  line L6 (-0.8394, 4.5479) -> (6.564, 4.5479)
  line L7 (6.564, 4.5479) -> (6.564, 2.6398)
  line L8 (9.6743, -1.4626) -> (-1.0111, -1.4626)
  line L9 (-1.0111, -1.4626) -> (-1.0111, 1.514)
  line L10 (-1.0111, 1.514) -> (9.6743, 1.514)
  line L11 (9.6743, 1.514) -> (9.6743, -1.4626)
  line L12 (-3.5996, -3.6349) -> (-1.0757, -3.6349)
  line L13 (-1.0757, -3.6349) -> (-1.0757, -7.7726)
  line L14 (-1.0757, -7.7726) -> (-3.5996, -7.7726)
  line L15 (-3.5996, -7.7726) -> (-3.5996, -3.6349)
  point P0 (-16, -32.4429)
  constraints: 32 end point, 8 parallel, 4 horizontal, 4 perpendicular
extrude "Wyciągnięcie proste41" cut sketch "Szkic47" against normal blind 2
sketch "Szkic48" plane through (-14, -12.0571, -8.5) normal (0, -1, 0) x (1, 0, 0)
  line L0 (7.8356, 0) -> (0, 0) projected
  line L1 (20, 0) -> (7.8356, 0) projected
  line L2 (20, 0) -> (0, -1.4964)
  line L3 (0, -1.4964) -> (0, 0)
  point P0 (14, 8.5)
  constraints: 4 end point, 1 perpendicular
extrude "Wyciągnięcie proste42" add sketch "Szkic48" against normal up to surface (50 mm away)
sketch "Szkic49" plane through (0, 37.9429, 10.5) normal (0, 1, 0) x (1, 0, 0)
  arc A0 (-6.1644, 19) -> (0, 0) centre (0, 10.5) ccw projected
  circle A1 centre (0, 10.5) radius 10.5
  line L0 (4.4, -19.3676) -> (6, -19.3676) projected
  line L1 (6, 0) -> (6, -19.3676) projected
  line L2 (0, 0) -> (6, 0) projected
  arc A2 (-6.1644, 19) -> (0, 0) centre (0, 10.5) ccw projected
  line L3 (6, 19) -> (-6.1644, 19) projected
  line L4 (-14, 20.4964) -> (6, 19) projected
  line L5 (-14, -22.771) -> (-14, 20.4964) projected
  line L6 (-14, -22.771) -> (4.4, -26.3676) projected
  line L7 (4.4, -26.3676) -> (4.4, -19.3676) projected
  point P0 (0, 10.5)
  point P1 (-4.8516, 19.8119)
  constraints: 1 centre point, 1 coincident
extrude "Wyciągnięcie proste43" cut sketch "Szkic49" against normal up to surface (7.533 mm away) contours A1 L4 L3
sketch "Szkic50" plane through (-14, -12.0571, 6) normal (0, -1, 0) x (1, 0, 0)
  line L0 (5.3832, 0) -> (0, 0) projected
  line L1 (0, 0) -> (0, -15.9964) projected
  line L2 (0, -15.9964) -> (20, -14.5) projected
  line L3 (20, -14.5) -> (7.8356, -14.5) projected
  arc A0 (5.3832, 0) -> (7.8356, -14.5) centre (14, -6) ccw projected
  arc A1 (5.3832, 0) -> (7.8356, -14.5) centre (14, -6) ccw projected
  circle A2 centre (14, -6) radius 10.5
  point P0 (9.1484, -15.3119)
  constraints: 1 coincident, 3 other
extrude "Wyciągnięcie proste44" cut sketch "Szkic50" against normal up to surface (12.0571 mm away) contours L3 L2 A2
